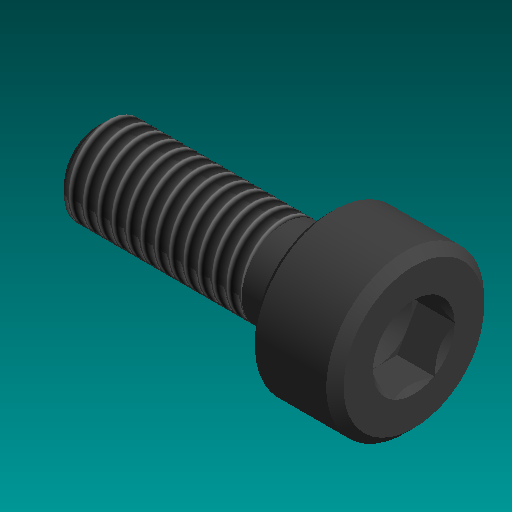
# Autodesk Inventor part: ISO-4762 M3x8
Saved by Autodesk Inventor 2020.3 (Build 243373000, 373)
## iProperties
Part Number: ISO-4762 M3x8
Material: Generic
Catalog Web Link: www.cadenas.de
Description: ISO-4762-Cylinder head screws cap screws
Vendor: FESTO
Document SubType Name: Modeling
Designer: partserver
Manufacturer: FESTO
Mass: 0.118757 g
Surface Area: 1.77239 cm^2
Volume: 0.118757 cm^3
Density: 1 g/cm^3
Appearance: PSOLRGB-80-80-80
Category: PARTsolutions
Company: FESTO
PSOL_IDENT_0: {$CADENAS_DATA\23d-libs\festo\zyl_zubeh\din_4762\din_en_iso_4762.prj},182 {VTYP=3D},{NB=ISO-4762 M3x
PSOL_IDENT_1: 8},{LINA=ISO-4762 M3x8},{NN=ISO-4762},{DATE=19.05.2020 13:42:07},{GEOMDATE=17.07.2018 07:56:43},{VER
PSOL_IDENT_2: SION=v080331135824},{LINEID=300},{WBVAR=},{WBNUMERIC=}  {NB=ISO-4762 M3x8},{LINA=ISO-4762 M3x8},{KT=
PSOL_IDENT_3: DUMMY},{IDNR=},{D=3.000},{D3=2.387},{P=0.500},{L=8.000},{B=6.5},{BX=18.000},{LS=0},{LG=1.5},{DK=5.50
PSOL_IDENT_4: 0},{DA=3.600},{DS=3.000},{E=2.870},{LF=0.510},{K=3.000},{R=0.100},{S=2.500},{T=1.300},{V=0.300},{DW=
PSOL_IDENT_5: 5.070},{W=1.150},{NENN=M3x8}
NB: ISO-4762 M3x8
NN: ISO-4762
NT: Cylinder head screws cap screws
NBSYN: ISO-4762 $NENN.
LINA: ISO-4762 M3x8
CATALOG: Festo
ROWDESC: M3x8
D: 3
D3: 2.387
P: 0.5
L: 8
B: 6.5
LS: 0
LG: 1.5
DK: 5.5
DA: 3.6
DS: 3
E: 2.87
LF: 0.51
K: 3
R: 0.1
S: 2.5
T: 1.3
V: 0.3
DW: 5.07
W: 1.15
SUPPLIER: FESTO
ARTICLENO: ISO-4762 M3x8
BOMINFO: ISO-4762 M3x8
CREATOR: CADENAS GmbH
Title: ISO-4762 M3x8
Author: Cadenas PARTsolutions
Comments: Cylinder head screws cap screws
Autodesk Inventor part; units mm, degrees
sketch "Sketch_1" plane through (0, 0, 0) normal (0, 0, 1) x (1, 0, 0)
  line L0 (8, 0) -> (-3, 0)
  line L1 (-3, 0) -> (-3, 2.75)
  line L2 (-3, 2.75) -> (0, 2.75)
  line L3 (0, 2.75) -> (0, 1.8)
  line L4 (0, 1.8) -> (0.51, 1.5)
  line L5 (0.51, 1.5) -> (7.6935, 1.5)
  line L6 (7.6935, 1.5) -> (8, 1.1935)
  line L7 (8, 1.1935) -> (8, 0)
  line L8 (8, 0) -> (-3, 0)
  constraints: 18 end point
revolve "Revolution1" add sketch "Sketch_1" angle 360 about axis through (8, 0, 0) along (1, 0, 0)
thread "Thread1" size "M3x0.5" class "6g" standard "ISO Metric profile" length 6.1935
sketch "Sketch_6" plane through (0, 0, 0) normal (0, 0, 1) x (1, 0, 0)
  line L0 (0, 0) -> (-3, 0)
  line L1 (-3, 3.3) -> (-3, 2.45)
  line L2 (-3, 2.45) -> (-2.7, 2.75)
  line L3 (-2.7, 2.75) -> (-0.215, 2.75)
  line L4 (-0.215, 2.75) -> (0, 2.535)
  line L5 (0, 2.535) -> (0, 3.3)
  line L6 (0, 3.3) -> (-3, 3.3)
  constraints: 14 end point
revolve "Revolution2" cut sketch "Sketch_6" angle 360 about axis through (0, 0, 0) along (1, 0, 0)
sketch "Sketch3" plane through (-3, 0, 0) normal (-1, 0, 0) x (0, 0, 1)
  point P0 (0, 0)
hole "Hole1" at (-3, 0, 0) direction (1, 0, 0) diameter 2.5 depth 1.3 tip angle 120 countersink diameter 2.85 countersink angle 90
sketch "Sketch_2" plane through (-3, 0, 0) normal (1, 0, 0) x (0, 0, -1)
  line L0 (-1.25, -0.7217) -> (0, -1.4434)
  line L1 (0, -1.4434) -> (1.25, -0.7217)
  line L2 (1.25, -0.7217) -> (1.25, 0.7217)
  line L3 (1.25, 0.7217) -> (0, 1.4434)
  line L4 (0, 1.4434) -> (-1.25, 0.7217)
  line L5 (-1.25, 0.7217) -> (-1.25, -0.7217)
  constraints: 12 end point
extrude "Extrusion1" cut sketch "Sketch_2" along normal mid plane 2.6
ref_plane "ANBAU_XY" through (0, 0, 0) normal (-1, 0, 0) x (0, 0, -1)
ref_plane "ANBAU_YZ" through (0, 0, 0) normal (0, 0, -1) x (0, -1, 0)
ref_plane "ANBAU_ZX" through (0, 0, 0) normal (0, -1, 0) x (-1, 0, 0)
ref_plane "IP1_XY" through (0, 0, 0) normal (1, 0, 0) x (0, 0, -1)
ref_plane "IP1_YZ" through (0, 0, 0) normal (0, 0, -1) x (0, 1, 0)
ref_plane "IP1_ZX" through (0, 0, 0) normal (0, 1, 0) x (1, 0, 0)
ref_plane "IP2_XY" through (-3, 0, 0) normal (1, 0, 0) x (0, 0, -1)
ref_plane "IP2_YZ" through (-3, 0, 0) normal (0, 0, -1) x (0, 1, 0)
ref_plane "IP2_ZX" through (-3, 0, 0) normal (0, 1, 0) x (1, 0, 0)
ref_plane "IP3_XY" through (8, 0, 0) normal (1, 0, 0) x (0, 0, -1)
ref_plane "IP3_YZ" through (8, 0, 0) normal (0, 0, -1) x (0, 1, 0)
ref_plane "IP3_ZX" through (8, 0, 0) normal (0, 1, 0) x (1, 0, 0)
body "Solid1"
